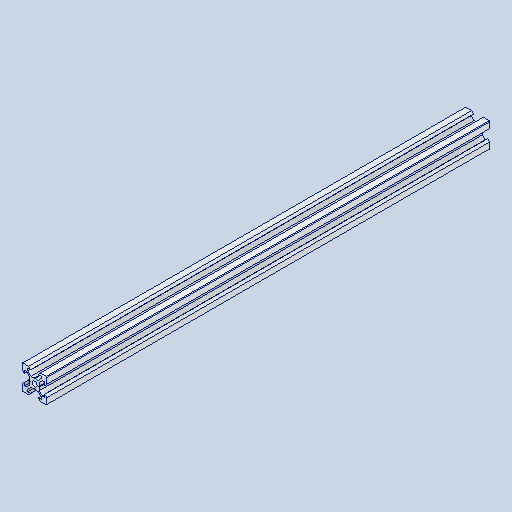
# Autodesk Inventor part: v-slot
Saved by Autodesk Inventor 2025.1 (Build 291241000, 241)
## iProperties
Created: 2024-09-08
Part Number: v-slot
Material: Aluminum 6061
Document SubType Name: Modeling
Designer: joser
Density: 2.7 g/cm^3
Appearance: Aluminum - Flat
Author: joser
Autodesk Inventor part; units mm, degrees
ref_plane "YZ Plane" through (0, 0, 0) normal (1, 0, 0) x (0, 1, 0)
ref_plane "XZ Plane" through (0, 0, 0) normal (0, 1, 0) x (-1, 0, 0)
ref_plane "XY Plane" through (0, 0, 0) normal (0, 0, 1) x (1, 0, 0)
sketch "Sketch2" plane through (0, 0, 0) normal (0, 0, 1) x (1, 0, 0)
  arc A0 (-27.4375, 16.3608) -> (-26.9375, 16.8608) centre (-27.4375, 16.8608) ccw
  line L0 (-45.4375, 36.3608) -> (-46.4375, 36.3608)
  line L1 (-46.9375, 34.8608) -> (-46.9375, 35.8608)
  line L2 (-28.4375, 36.3608) -> (-27.4375, 36.3608)
  line L3 (-26.9375, 17.8608) -> (-26.9375, 16.8608)
  line L4 (-28.4375, 16.3608) -> (-27.4375, 16.3608)
  line L5 (-26.9375, 31.1923) -> (-26.9375, 35.8608)
  line L6 (-46.4375, 16.3608) -> (-41.7689, 16.3608)
  line L7 (-46.9375, 17.8608) -> (-46.9375, 16.8608)
  arc A1 (-46.9375, 16.8608) -> (-46.4375, 16.3608) centre (-46.4375, 16.8608) ccw
  arc A2 (-46.9375, 16.8608) -> (-46.4375, 16.3608) centre (-46.4375, 16.8608) ccw
  arc A3 (-46.4375, 36.3608) -> (-46.9375, 35.8608) centre (-46.4375, 35.8608) ccw
  arc A4 (-26.9375, 35.8608) -> (-27.4375, 36.3608) centre (-27.4375, 35.8608) ccw
  line L8 (-41.5004, 36.2982) -> (-41.5366, 36.3146)
  line L9 (-46.812, 30.8227) -> (-46.8352, 30.855)
  line L10 (-46.9375, 17.8608) -> (-46.9375, 21.4608)
  line L11 (-46.9362, 21.5691) -> (-46.9375, 21.4608)
  line L12 (-46.9258, 21.6478) -> (-46.9323, 21.6086)
  line L13 (-46.9323, 21.6086) -> (-46.9362, 21.5691)
  line L14 (-46.9168, 21.6865) -> (-46.9258, 21.6478)
  line L15 (-46.9053, 21.7245) -> (-46.9168, 21.6865)
  line L16 (-46.8913, 21.7617) -> (-46.9053, 21.7245)
  line L17 (-46.8749, 21.7979) -> (-46.8913, 21.7617)
  line L18 (-46.8561, 21.8329) -> (-46.8749, 21.7979)
  line L19 (-46.812, 21.8989) -> (-46.8352, 21.8667)
  line L20 (-46.8352, 21.8667) -> (-46.8561, 21.8329)
  line L21 (-41.4654, 36.2795) -> (-41.5004, 36.2982)
  line L22 (-46.7868, 21.9297) -> (-46.812, 21.8989)
  line L23 (-46.7597, 21.9586) -> (-46.7868, 21.9297)
  line L24 (-46.7597, 21.9586) -> (-45.2441, 23.4742)
  line L25 (-45.2441, 23.4742) -> (-45.1375, 23.4742)
  line L26 (-45.1375, 23.4742) -> (-45.1375, 20.8608)
  line L27 (-45.1375, 20.8608) -> (-43.4981, 20.8608)
  line L28 (-43.4981, 20.8608) -> (-40.8375, 23.5215)
  line L29 (-46.7868, 30.792) -> (-46.812, 30.8227)
  line L30 (-40.8375, 26.161) -> (-40.8375, 23.5215)
  line L31 (-40.6376, 26.3608) -> (-40.8375, 26.161)
  line L32 (-40.6376, 26.3608) -> (-40.8375, 26.5607)
  line L33 (-40.8375, 29.2002) -> (-40.8375, 26.5607)
  line L34 (-43.4981, 31.8608) -> (-40.8375, 29.2002)
  line L35 (-45.1375, 31.8608) -> (-43.4981, 31.8608)
  line L36 (-45.1375, 29.2475) -> (-45.1375, 31.8608)
  line L37 (-46.7597, 30.763) -> (-46.7868, 30.792)
  line L38 (-45.2441, 29.2475) -> (-45.1375, 29.2475)
  line L39 (-45.2441, 29.2475) -> (-46.7597, 30.763)
  line L40 (-28.7375, 20.8608) -> (-30.3768, 20.8608)
  line L41 (-41.5738, 36.3286) -> (-41.6118, 36.3402)
  line L42 (-41.3687, 36.2102) -> (-41.3994, 36.2354)
  line L43 (-41.3397, 36.183) -> (-41.3687, 36.2102)
  line L44 (-41.6118, 36.3402) -> (-41.6505, 36.3492)
  line L45 (-41.7292, 16.3621) -> (-41.7689, 16.3608)
  line L46 (-41.6897, 16.366) -> (-41.7292, 16.3621)
  line L47 (-41.6505, 16.3725) -> (-41.6897, 16.366)
  line L48 (-41.6118, 16.3815) -> (-41.6505, 16.3725)
  line L49 (-41.5738, 16.3931) -> (-41.6118, 16.3815)
  line L50 (-41.5366, 16.4071) -> (-41.5738, 16.3931)
  line L51 (-42.4375, 32.9215) -> (-39.7768, 30.2608)
  line L52 (-41.5004, 16.4235) -> (-41.5366, 16.4071)
  line L53 (-41.4654, 16.4422) -> (-41.5004, 16.4235)
  line L54 (-41.4317, 16.4632) -> (-41.4654, 16.4422)
  line L55 (-41.3994, 16.4863) -> (-41.4317, 16.4632)
  line L56 (-41.3687, 16.5115) -> (-41.3994, 16.4863)
  line L57 (-41.3397, 16.5386) -> (-41.3687, 16.5115)
  line L58 (-41.3397, 16.5386) -> (-39.8241, 18.0542)
  line L59 (-39.8241, 18.0542) -> (-39.8241, 18.1608)
  line L60 (-39.8241, 18.1608) -> (-42.4375, 18.1608)
  line L61 (-42.4375, 18.1608) -> (-42.4375, 19.8002)
  line L62 (-42.4375, 19.8002) -> (-39.7768, 22.4608)
  line L63 (-39.7768, 22.4608) -> (-37.1444, 22.4608)
  line L64 (-37.1444, 22.4608) -> (-36.9375, 22.6656)
  line L65 (-36.9375, 22.6656) -> (-36.7327, 22.4608)
  line L66 (-36.7327, 22.4608) -> (-34.0981, 22.4608)
  line L67 (-34.0981, 22.4608) -> (-31.4375, 19.8002)
  line L68 (-31.4375, 18.1608) -> (-31.4375, 19.8002)
  line L69 (-41.3397, 36.183) -> (-39.8241, 34.6675)
  line L70 (-34.0508, 18.1608) -> (-31.4375, 18.1608)
  line L71 (-41.6505, 36.3492) -> (-41.6897, 36.3557)
  line L72 (-34.0508, 18.0542) -> (-34.0508, 18.1608)
  line L73 (-34.0508, 18.0542) -> (-32.5353, 16.5387)
  line L74 (-32.5353, 16.5387) -> (-32.5063, 16.5115)
  line L75 (-32.5063, 16.5115) -> (-32.4756, 16.4863)
  line L76 (-32.4756, 16.4863) -> (-32.4433, 16.4632)
  line L77 (-32.4433, 16.4632) -> (-32.4096, 16.4422)
  line L78 (-32.4096, 16.4422) -> (-32.3745, 16.4235)
  line L79 (-32.3745, 16.4235) -> (-32.3383, 16.4071)
  line L80 (-32.3383, 16.4071) -> (-32.3012, 16.3931)
  line L81 (-32.3012, 16.3931) -> (-32.2631, 16.3815)
  line L82 (-32.2631, 16.3815) -> (-32.2245, 16.3725)
  line L83 (-32.2245, 16.3725) -> (-32.1853, 16.366)
  line L84 (-32.1853, 16.366) -> (-32.1457, 16.3621)
  line L85 (-32.1457, 16.3621) -> (-32.106, 16.3608)
  line L86 (-28.4375, 16.3608) -> (-32.106, 16.3608)
  line L87 (-39.8241, 34.6675) -> (-39.8241, 34.5608)
  line L88 (-41.6897, 36.3557) -> (-41.7292, 36.3595)
  line L89 (-26.9375, 17.8608) -> (-26.9375, 21.5294)
  line L90 (-26.9388, 21.5691) -> (-26.9375, 21.5294)
  line L91 (-26.9427, 21.6086) -> (-26.9388, 21.5691)
  line L92 (-26.9491, 21.6478) -> (-26.9427, 21.6086)
  line L93 (-26.9582, 21.6865) -> (-26.9491, 21.6478)
  line L94 (-26.9697, 21.7245) -> (-26.9582, 21.6865)
  line L95 (-26.9837, 21.7617) -> (-26.9697, 21.7245)
  line L96 (-27.0001, 21.7979) -> (-26.9837, 21.7617)
  line L97 (-41.7292, 36.3595) -> (-41.7689, 36.3608)
  line L98 (-27.0188, 21.8329) -> (-27.0001, 21.7979)
  line L99 (-27.0398, 21.8667) -> (-27.0188, 21.8329)
  line L100 (-27.0629, 21.8989) -> (-27.0398, 21.8667)
  line L101 (-27.0881, 21.9297) -> (-27.0629, 21.8989)
  line L102 (-27.1153, 21.9587) -> (-27.0881, 21.9297)
  line L103 (-28.6308, 23.4742) -> (-27.1153, 21.9587)
  line L104 (-28.6308, 23.4742) -> (-28.7375, 23.4742)
  line L105 (-28.7375, 23.4742) -> (-28.7375, 20.8608)
  line L106 (-32.3012, 36.3286) -> (-32.2631, 36.3402)
  line L107 (-30.3768, 20.8608) -> (-33.0375, 23.5215)
  line L108 (-33.0375, 23.5215) -> (-33.0375, 26.161)
  line L109 (-33.2373, 26.3608) -> (-33.0375, 26.161)
  line L110 (-33.2373, 26.3608) -> (-33.0375, 26.5607)
  line L111 (-33.0375, 29.2002) -> (-33.0375, 26.5607)
  line L112 (-30.3768, 31.8608) -> (-33.0375, 29.2002)
  line L113 (-45.4375, 36.3608) -> (-41.7689, 36.3608)
  line L114 (-28.6308, 29.2475) -> (-28.7375, 29.2475)
  line L115 (-28.7375, 31.8608) -> (-30.3768, 31.8608)
  line L116 (-28.7375, 29.2475) -> (-28.7375, 31.8608)
  line L117 (-27.1153, 30.763) -> (-28.6308, 29.2475)
  line L118 (-27.1153, 30.763) -> (-27.0881, 30.792)
  line L119 (-27.0881, 30.792) -> (-27.0629, 30.8227)
  line L120 (-27.0629, 30.8227) -> (-27.0398, 30.855)
  line L121 (-27.0398, 30.855) -> (-27.0188, 30.8888)
  line L122 (-27.0188, 30.8888) -> (-27.0001, 30.9238)
  line L123 (-27.0001, 30.9238) -> (-26.9837, 30.96)
  line L124 (-26.9837, 30.96) -> (-26.9697, 30.9972)
  line L125 (-26.9697, 30.9972) -> (-26.9582, 31.0352)
  line L126 (-26.9582, 31.0352) -> (-26.9491, 31.0739)
  line L127 (-26.9491, 31.0739) -> (-26.9427, 31.1131)
  line L128 (-26.9427, 31.1131) -> (-26.9388, 31.1526)
  line L129 (-26.9388, 31.1526) -> (-26.9375, 31.1923)
  line L130 (-39.8241, 34.5608) -> (-42.4375, 34.5608)
  line L131 (-28.4375, 36.3608) -> (-32.106, 36.3608)
  line L132 (-32.1457, 36.3595) -> (-32.106, 36.3608)
  line L133 (-32.1853, 36.3557) -> (-32.1457, 36.3595)
  line L134 (-32.2631, 36.3402) -> (-32.2245, 36.3492)
  line L135 (-32.3383, 36.3146) -> (-32.3012, 36.3286)
  line L136 (-32.3745, 36.2982) -> (-32.3383, 36.3146)
  line L137 (-32.4096, 36.2795) -> (-32.3745, 36.2982)
  line L138 (-32.4433, 36.2585) -> (-32.4096, 36.2795)
  line L139 (-32.4756, 36.2354) -> (-32.4433, 36.2585)
  line L140 (-32.5063, 36.2102) -> (-32.4756, 36.2354)
  line L141 (-46.9323, 31.1131) -> (-46.9362, 31.1526)
  line L142 (-34.0508, 34.6675) -> (-32.5353, 36.183)
  line L143 (-34.0508, 34.6675) -> (-34.0508, 34.5608)
  line L144 (-34.0508, 34.5608) -> (-31.4375, 34.5608)
  line L145 (-31.4375, 34.5608) -> (-31.4375, 32.9215)
  line L146 (-34.0981, 30.2608) -> (-31.4375, 32.9215)
  line L147 (-34.0981, 30.2608) -> (-36.7327, 30.2608)
  line L148 (-42.4375, 34.5608) -> (-42.4375, 32.9215)
  line L149 (-36.7327, 30.2608) -> (-36.9375, 30.0561)
  line L150 (-37.1422, 30.2608) -> (-36.9375, 30.0561)
  line L151 (-39.7768, 30.2608) -> (-37.1422, 30.2608)
  line L152 (-32.5353, 36.183) -> (-32.5063, 36.2102)
  line L153 (-41.3994, 36.2354) -> (-41.4317, 36.2585)
  line L154 (-46.9258, 31.0739) -> (-46.9323, 31.1131)
  line L155 (-41.4317, 36.2585) -> (-41.4654, 36.2795)
  line L156 (-46.9362, 31.1526) -> (-46.9375, 31.2608)
  line L157 (-46.9168, 31.0352) -> (-46.9258, 31.0739)
  line L158 (-46.9375, 34.8608) -> (-46.9375, 31.2608)
  line L159 (-46.9053, 30.9972) -> (-46.9168, 31.0352)
  line L160 (-46.8913, 30.96) -> (-46.9053, 30.9972)
  line L161 (-46.8749, 30.9238) -> (-46.8913, 30.96)
  line L162 (-46.8561, 30.8888) -> (-46.8749, 30.9238)
  line L163 (-32.2245, 36.3492) -> (-32.1853, 36.3557)
  line L164 (-41.5366, 36.3146) -> (-41.5738, 36.3286)
  line L165 (-46.8352, 30.855) -> (-46.8561, 30.8888)
  circle A5 centre (-36.9375, 26.3608) radius 2.1
  line L166 (3.9, -0.3) -> (3.9, -2.8393)
  line L167 (2.8393, -3.9) -> (0.3, -3.9)
  line L168 (5.5, -6.5607) -> (2.8393, -3.9)
  line L169 (3.9, -2.8393) -> (6.5607, -5.5)
  line L170 (6.5607, -5.5) -> (8.2007, -5.5)
  line L171 (8.2007, -5.5) -> (8.2007, -3.125)
  line L172 (8.2007, -3.125) -> (8.4007, -3.125)
  line L173 (8.4007, -3.125) -> (10.0007, -4.725)
  line L174 (10.0007, -9.5007) -> (10.0007, -4.725)
  line L175 (5.5, -6.5607) -> (5.5, -8.2007)
  line L176 (5.5, -8.2007) -> (3.125, -8.2007)
  line L177 (3.125, -8.2007) -> (3.125, -8.4007)
  line L178 (3.125, -8.4007) -> (4.725, -10.0007)
  line L179 (9.5007, -10.0007) -> (4.725, -10.0007)
  arc A6 (9.5007, -10.0007) -> (10.0007, -9.5007) centre (9.5007, -9.5007) ccw
  line L180 (0, -3.6) -> (0.3, -3.9)
  line L181 (3.6, 0) -> (3.9, -0.3)
  line L182 (3.125, 8.2007) -> (3.125, 8.4007)
  line L183 (0.3, 3.9) -> (2.8393, 3.9)
  line L184 (5.5, 8.2007) -> (3.125, 8.2007)
  line L185 (2.8393, 3.9) -> (5.5, 6.5607)
  line L186 (3.9, 2.8393) -> (3.9, 0.3)
  line L187 (3.6, 0) -> (3.9, 0.3)
  line L188 (6.5607, 5.5) -> (3.9, 2.8393)
  line L189 (5.5, 6.5607) -> (5.5, 8.2007)
  line L190 (3.125, 8.4007) -> (4.725, 10.0007)
  line L191 (6.5607, 5.5) -> (8.2007, 5.5)
  line L192 (8.2007, 5.5) -> (8.2007, 3.125)
  line L193 (8.2007, 3.125) -> (8.4007, 3.125)
  line L194 (8.4007, 3.125) -> (10.0007, 4.725)
  line L195 (9.5007, 10.0007) -> (4.725, 10.0007)
  arc A7 (10.0007, 9.5007) -> (9.5007, 10.0007) centre (9.5007, 9.5007) ccw
  line L196 (10.0007, 9.5007) -> (10.0007, 4.725)
  line L197 (0, 3.6) -> (0.3, 3.9)
  line L198 (-8.2007, 3.125) -> (-8.4007, 3.125)
  line L199 (-3.9, 0.3) -> (-3.9, 2.8393)
  line L200 (-8.2007, 5.5) -> (-8.2007, 3.125)
  line L201 (-3.9, 2.8393) -> (-6.5607, 5.5)
  line L202 (-2.8393, 3.9) -> (-0.3, 3.9)
  line L203 (0, 3.6) -> (-0.3, 3.9)
  line L204 (-5.5, 6.5607) -> (-2.8393, 3.9)
  line L205 (-6.5607, 5.5) -> (-8.2007, 5.5)
  line L206 (-8.4007, 3.125) -> (-10.0007, 4.725)
  line L207 (-5.5, 6.5607) -> (-5.5, 8.2007)
  line L208 (-5.5, 8.2007) -> (-3.125, 8.2007)
  line L209 (-3.125, 8.2007) -> (-3.125, 8.4007)
  line L210 (-3.125, 8.4007) -> (-4.725, 10.0007)
  line L211 (-10.0007, 9.5007) -> (-10.0007, 4.725)
  arc A8 (-9.5007, 10.0007) -> (-10.0007, 9.5007) centre (-9.5007, 9.5007) ccw
  line L212 (-9.5007, 10.0007) -> (-4.725, 10.0007)
  line L213 (-3.6, 0) -> (-3.9, 0.3)
  line L214 (-3.125, -8.2007) -> (-3.125, -8.4007)
  line L215 (-0.3, -3.9) -> (-2.8393, -3.9)
  line L216 (-5.5, -8.2007) -> (-3.125, -8.2007)
  line L217 (-2.8393, -3.9) -> (-5.5, -6.5607)
  line L218 (-3.9, -2.8393) -> (-3.9, -0.3)
  line L219 (-3.6, 0) -> (-3.9, -0.3)
  line L220 (-6.5607, -5.5) -> (-3.9, -2.8393)
  line L221 (-5.5, -6.5607) -> (-5.5, -8.2007)
  line L222 (-3.125, -8.4007) -> (-4.725, -10.0007)
  line L223 (-6.5607, -5.5) -> (-8.2007, -5.5)
  line L224 (-8.2007, -5.5) -> (-8.2007, -3.125)
  line L225 (-8.2007, -3.125) -> (-8.4007, -3.125)
  line L226 (-8.4007, -3.125) -> (-10.0007, -4.725)
  line L227 (-9.5007, -10.0007) -> (-4.725, -10.0007)
  arc A9 (-10.0007, -9.5007) -> (-9.5007, -10.0007) centre (-9.5007, -9.5007) ccw
  line L228 (-10.0007, -9.5007) -> (-10.0007, -4.725)
  line L229 (0, -3.6) -> (-0.3, -3.9)
  circle A10 centre (0, 0) radius 2.1
  point P0 (0, -3.9)
  point P1 (3.9, 0)
  point P2 (3.9, 0)
  point P3 (0, 3.9)
  point P4 (0, 3.9)
  point P5 (3.9, 0)
  point P6 (-3.9, 0)
  point P7 (-3.9, 0)
  point P8 (0, 3.9)
  point P9 (0, -3.9)
  point P10 (0, -3.9)
  point P11 (-3.9, 0)
  dimension "d1" = 4.2
  dimension "d2" = 1.5
  dimension "d4" = 3.9
  dimension "d5" = 3.9
  dimension "d7" = 1.5
  dimension "d9" = 1.64
  dimension "d10" = 135
  dimension "d11" = 1.8
  dimension "d12" = 3.125
  dimension "d13" = 5.5
  dimension "d14" = 45
  dimension "d15" = 0.2
  dimension "d16" = 0.5
  dimension "d17" = 0.3
  dimension "d18" = 0.3
  dimension "d19" = 0.3
  dimension "d20" = 0.3
  dimension "d23" = 360
  dimension "d25" = 4.2
  constraints: 460 end point, 18 point on circle, 12 point on line, 11 centre point, 3 coincident, 3 vertical, 2 horizontal, 2 tangent, 1 parallel, 1 perpendicular, 157 other
  measures "d1" diameter of A5
  measures "d2" distance between parallel lines of L62 L28
  measures "d4" distance from line of point (0, 0) L166
  measures "d5" distance from line of point (0, 0) L167
  measures "d7" distance between parallel lines of L169 L168
  measures "d9" distance of L169.end L170.end
  measures "d10" angle of L172 L173
  measures "d11" distance between parallel lines of L174 L171
  measures "d12" distance from line of point (0, 0) L172
  measures "d13" distance from line of point (0, 0) L170
  measures "d14" angle of L169 L166
  measures "d15" distance of L171.end L172.end
  measures "d16" radius of A6
  measures "d17" distance of L180.start point (0, -3.9)
  measures "d18" distance of L167.end point (0, -3.9)
  measures "d19" distance of L181.start point (3.9, 0)
  measures "d20" distance of L166.start point (3.9, 0)
  measures "d25" diameter of A10
extrude "Extrusion1" add sketch "Sketch2" against normal blind 360 contours L166 L169 L170 L171 L172 L173 L174 A6 L179 L178 L177 L176 L175 L168 L167 L180 L229 L215 L217 L221 L216 L214 L222 L227 A9 L228 L226 L225 L224 L223 L220 L218 L219 L213 L199 L201 L205 L200 L198 L206 L211 A8 L212 L210 L209 L208 L207 L204 L202 L203 L197 L183 L185 L189 L184 L182 L190 L195 A7 L196 L194 L193 L192 L191 L188 L186 L187 L181
equation "\"d5\" = d4"
equation "\"d18\" = d17"
equation "\"d20\" = d19"
body "Solid1"
